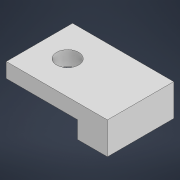
# Autodesk Inventor part: gear support attachment
Saved by Autodesk Inventor 2022 (Build 260153000, 153)
## iProperties
Created: 2022-01-26
Part Number: gear support attachment
Material: Generic
Document SubType Name: Modeling
Designer: gordo
Density: 1 g/cm^3
Appearance: Default
Author: gordo
Autodesk Inventor part; units mm, degrees
ref_plane "YZ Plane" through (0, 0, 0) normal (1, 0, 0) x (0, 1, 0)
ref_plane "XZ Plane" through (0, 0, 0) normal (0, 1, 0) x (-1, 0, 0)
ref_plane "XY Plane" through (0, 0, 0) normal (0, 0, 1) x (1, 0, 0)
sketch "Sketch1" plane through (0, 0, 0) normal (1, 0, 0) x (0, 1, 0)
  line L0 (0, 0) -> (6.5, 0)
  line L1 (6.5, 0) -> (6.5, -13.5)
  line L2 (6.5, -13.5) -> (0, -13.5)
  line L3 (0, -13.5) -> (0, 0)
  dimension "d0" = 6.5
  dimension "d1" = 13.5
  constraints: 8 end point, 2 parallel, 1 horizontal, 1 perpendicular
  measures "d0" distance between parallel lines of L1 L3
  measures "d1" distance between parallel lines of L2 L0
extrude "Extrusion1" add sketch "Sketch1" along normal blind 6.1
sketch "Sketch2" plane through (0, 0, 0) normal (-1, 0, 0) x (0, 0, 1)
  line L0 (-13.5, 3.5) -> (0, 3.5)
  line L1 (0, 3.5) -> (0, 6.5)
  line L2 (0, 6.5) -> (-13.5, 6.5)
  line L3 (-13.5, 6.5) -> (-13.5, 3.5)
  line L4 (0, 6.5) -> (0, 0) projected
  line L5 (-13.5, 6.5) -> (0, 6.5) projected
  dimension "d4" = 3
  dimension "d5" = 13.5
  dimension "d6" = 0
  dimension "d7" = 0
  constraints: 8 end point, 2 parallel, 1 horizontal, 1 perpendicular
  measures "d4" distance between parallel lines of L0 L2
  measures "d5" distance between parallel lines of L1 L3
  measures "d6" distance between parallel lines of L4 L1
  measures "d7" distance between parallel lines of L5 L2
extrude "Extrusion2" add sketch "Sketch2" along normal blind 14.5
sketch "Sketch3" plane through (6.1, 6.5, 0) normal (0, 1, 0) x (1, 0, 0)
  circle A0 centre (-14.85, 6.75) radius 2.25
  line L0 (-20.6, 0) -> (-20.6, 13.5) projected
  line L1 (-20.6, 0) -> (0, 0) projected
  point P0 (-6.1, 0)
  dimension "d10" = 4.5
  dimension "d11" = 5.75
  dimension "d12" = 6.75
  constraints: 1 centre point
  measures "d10" diameter of A0
  measures "d11" distance from line of L0 A0.centre
  measures "d12" distance from line of L1 A0.centre
extrude "Extrusion3" cut sketch "Sketch3" against normal blind 14.5
sketch "Sketch4" plane through (6.1, 0, -13.5) normal (0, 0, -1) x (-1, 0, 0)
  point P0 (6.1, 0)
body "Solid1"
